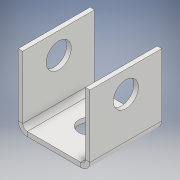
# Autodesk Inventor part: Ground_Tracker_Bearing
Saved by Autodesk Inventor 2018 (Build 220112000, 112)
## iProperties
Created: 2018-09-27
Part Number: Ground_Tracker_Bearing
Material: UHMW, White
Document SubType Name: Sheet Metal
Designer: Bradley
Density: 0.94 g/cm^3
Sheet Metal Rule: Default_mm
Appearance: Smooth - White
Author: Bradley
Autodesk Inventor part; units mm, degrees
ref_plane "YZ Plane" through (0, 0, 0) normal (1, 0, 0) x (0, 1, 0)
ref_plane "XZ Plane" through (0, 0, 0) normal (0, 1, 0) x (-1, 0, 0)
ref_plane "XY Plane" through (0, 0, 0) normal (0, 0, 1) x (1, 0, 0)
sketch "Sketch1" plane through (0, 0, 0) normal (0, 0, 1) x (1, 0, 0)
  line L0 (-50, -50) -> (50, -50)
  line L1 (50, -50) -> (50, 50)
  line L2 (50, 50) -> (-50, 50)
  line L3 (-50, 50) -> (-50, -50)
  line L4 (-50, -50) -> (50, 50) construction
  line L5 (50, -50) -> (-50, 50) construction
  point P0 (0, 0)
  dimension "d0" = 100
  dimension "d1" = 100
  measures "d0" distance of L2.end L1.end
  measures "d1" distance of L1.end L0.end
extrude "Plate1" add sketch "Sketch1" along normal blind 6.35
sketch "Sketch2" plane through (-43.65, -50, 0) normal (-1, 0, 0) x (0, -1, 0)
  line L0 (-100, 0) -> (0, 0)
  line L1 (0, 0) -> (0, 100)
  line L2 (0, 100) -> (-100, 100)
  line L3 (-100, 100) -> (-100, 0)
  constraints: 6 end point, 1 horizontal, 1 perpendicular, 1 vertical
edge flange "Flange1" height 100 angle 90 thickness 6.35 bend radius 6.35 thickness toward (-1, 0, 0) relief straight relief width 6.35 relief depth 3.175 corner gap 6.35 corner form 0 edges at (-50, 0, 6.35) (50, 0, 6.35) wall of the first edge with corners at (-43.65, 50, 0) (-43.65, -50, 0) (-43.65, -50, 100) (-43.65, 50, 100)
bend "Bend1"
corner "Corner1"
sketch "Sketch3" plane through (50, -50, 100) normal (1, 0, 0) x (0, 0, -1)
  circle A0 centre (30, 50) radius 16.7005 construction
  circle A1 centre (30, 50) radius 17.5
  point P0 (100, 50)
  dimension "d13" = 33.401
  dimension "d14" = 35
  dimension "d15" = 70
  constraints: 2 centre point, 1 coincident, 1 horizontal alignment
  measures "d13" diameter of A0
  measures "d14" diameter of A1
  measures "d15" distance of point (100, 50) A0.centre
extrude "Cut1" cut sketch "Sketch3" against normal through all
sketch "Sketch4" plane through (0, 0, 6.35) normal (0, 0, 1) x (1, 0, 0)
  circle A0 centre (0, 0) radius 15.5
  dimension "d18" = 31
  constraints: 1 centre point, 1 coincident
  measures "d18" diameter of A0
extrude "Cut2" cut sketch "Sketch4" against normal blind 6.35
equation "\"d16\" = Thickness"
equation "\"d19\" = Thickness"
equation "\"d2\" = Thickness"
equation "\"d3\" = BendReliefWidth"
equation "\"d4\" = BendReliefDepth"
equation "\"d5\" = MinimumRemnant"
equation "\"d6\" = TransitionRadius"
equation "\"d9\" = BendRadius"
equation "\"d10\" = CornerReliefSize"
equation "\"d11\" = GapSize"
equation "\"d12\" = JacobiRadiusSize"
equation "\"BendRadius\" = Thickness"
equation "\"BendReliefWidth\" = Thickness"
equation "\"BendReliefDepth\" = 0.5 * Thickness"
equation "\"CornerReliefSize\" = 4 * Thickness"
equation "\"MinimumRemnant\" = 2 * Thickness"
equation "\"TransitionRadius\" = BendRadius"
equation "\"JacobiRadiusSize\" = BendRadius"
equation "\"GapSize\" = Thickness"
equation "\"Thickness\" = 6.35"
body "Solid1"
